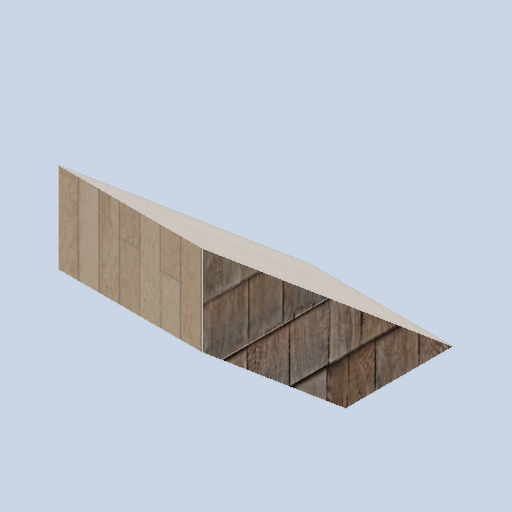
# Autodesk Inventor part: frame_rib_01
Saved by Autodesk Inventor 2024.2 (Build 282272000, 272)
## iProperties
Created: 2024-05-22
Part Number: frame_rib_01
Material: Wood (Maple)
Document SubType Name: Modeling
Designer: LOSTER_1
Density: 0.67 g/cm^3
Appearance: Natural Maple - Glossy Dark Tint
Author: LOSTER_1
Autodesk Inventor part; units mm, degrees
ref_plane "YZ Plane" through (0, 0, 0) normal (1, 0, 0) x (0, 1, 0)
ref_plane "XZ Plane" through (0, 0, 0) normal (0, 1, 0) x (-1, 0, 0)
ref_plane "XY Plane" through (0, 0, 0) normal (0, 0, 1) x (1, 0, 0)
sketch "Sketch1" plane through (0, 0, 0) normal (1, 0, 0) x (0, 1, 0)
  line L0 (-16157.1834, -1459.948) -> (-16157.1834, 1071.677)
  line L1 (-16157.1834, 1471.677) -> (-16157.1834, 1071.677)
  line L2 (-16157.1834, 1471.677) -> (-14157.1834, 1471.677)
  line L3 (-16157.1834, 1071.677) -> (-16157.1834, 771.677)
  line L4 (-16157.1834, 1071.677) -> (-15821.5435, 1471.677)
  line L5 (-16157.1834, 1071.677) -> (-15635.0204, 1071.677) construction
  line L6 (-16157.1834, 771.677) -> (-15569.8136, 1471.677)
  line L7 (-16157.1834, 771.677) -> (-15243.3983, 771.677) construction
  point P0 (0, 0)
  dimension "d2" = 300
  dimension "d11" = 50
  dimension "d12" = 50
  constraints: 16 end point, 3 point on line, 2 equal length, 2 horizontal
  measures "d2" distance of L0.end L3.end
  measures "d11" angle of L5 L4
  measures "d12" angle of L7 L6
extrude "Extrusion3" add sketch "Sketch1" along normal blind 400 contours L0 L4 L2 L6
body "Solid3"
